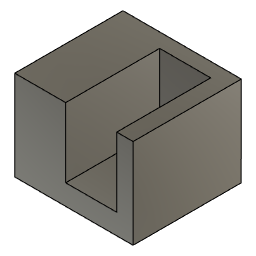
MotorHolder (Autodesk Fusion 360 design; units mm, degrees)
Autodesk Fusion 360 part; units mm, degrees
sketch "Sketch1" plane through (0, 0, 0) normal (0, 0, 1) x (1, 0, 0)
  line L0 (0, 0) -> (17, 0)
  line L1 (17, 0) -> (17, 23)
  line L2 (17, 23) -> (0, 23)
  line L3 (0, 23) -> (0, 0)
  dimension "d1" = 17
  dimension "d2" = 23
  constraint horizontal L0
  constraint vertical L1
  constraint horizontal L2
  constraint vertical L3
  constraint coincident L0.start L3.end
  measures "d1" distance of L0.start L0.end
  measures "d2" distance of L0.start L2.end
extrude "Extrude1" add sketch "Sketch1" along normal blind 3.5 makes body 1
sketch "Sketch2" plane through (0, 0, 3.5) normal (0, 0, 1) x (-1, 0, 0)
  line L0 (0, -23) -> (0, 0)
  line L1 (0, 0) -> (-17, 0)
  line L2 (-17, 0) -> (-17, -23)
  line L3 (-17, -23) -> (0, -23)
  line L4 (0, -25) -> (-17, -25)
  line L5 (-17, -25) -> (-17, -28.5)
  line L6 (-17, -28.5) -> (0, -28.5)
  line L7 (0, -28.5) -> (0, -25)
  dimension "d5" = 3.5
  constraint horizontal L4
  constraint vertical L5
  constraint horizontal L6
  constraint vertical L7
  measures "d5" distance of L4.start L6.end
extrude "Extrude2" add sketch "Sketch2" along normal blind 19 separate body contours L4 L5 L6 L7 makes body 2
copy_body "CopyPasteBodies1" bodies 1 makes body 3
move_body "Move1" bodies 3 to x (1, 0, 0) y (0, 1, 0) z (0, 0, 1) at (0, 0, 16)
move_body "Move2" bodies 2 to x (1, 0, 0) y (0, 1, 0) z (0, 0, 1) at (0, -2, -3.5)
move_body "Move3" bodies 3 to x (1, 0, 0) y (0, 1, 0) z (0, 0, 1) at (0, 0, -0.5)
sketch "Sketch3" plane through (0, 0, 0) normal (0, 1, 0) x (1, 0, 0)
sketch "Sketch4" plane through (0, 0, 0) normal (1, 0, 0) x (0, 1, 0)
  line L0 (26.467, 0.0177) -> (0, 0.0177)
  line L1 (0, 0.0177) -> (0, 19)
  line L2 (0, 19) -> (26.467, 19)
  line L3 (26.467, 19) -> (26.467, 0.0177)
  constraint horizontal L0
  constraint vertical L1
  constraint horizontal L2
  constraint vertical L3
move_body "Move4" bodies 3 2 1 to x (1, 0, 0) y (0, 1, 0) z (0, 0, 1) at (10, 0, 0)
extrude "Extrude3" add sketch "Sketch4" along normal blind 5 separate body makes body 4
move_body "Move5" bodies 4 to x (1, 0, 0) y (0, 1, 0) z (0, 0, 1) at (27, 0, 0)
combine "Combine1" operation add target body 2 tool bodies 3
combine "Combine2" operation add target body 2 tool bodies 1
combine "Combine3" operation add target body 4 tool bodies 2
move_body "Move6" bodies 4 to x (-1, 0, 0) y (0, 1, 0) z (0, 0, -1) at (56.1982, 0, 38)
move_body "Move7" bodies 4 to x (1, 0, 0) y (0, 1, 0) z (0, 0, 1) at (-19, 0, -19)
extrude "Extrude4" cut 1 faces at (21.5315, 15.3333, 3.5) along direction (0, 0, -1) blind 0.5 on bodies 4 bodies 4
extrude "Extrude5" cut 1 faces at (21.5315, 15.3333, 15.5) along direction (0, 0, 1) blind 0.5 on bodies 4 bodies 4
extrude "Extrude6" add 1 faces at (6.8648, 16.489, 18.9823) along direction (0, 0, 1) blind 10 on bodies 4 bodies 4
extrude "Extrude7" add 1 faces at (21.5315, 16.5, 19) along direction (0, 0, 1) blind 9.982 on bodies 4 bodies 4
move_body "Move8" bodies 4 to x (0, 0, 1) y (0, 1, 0) z (-1, 0, 0) at (43.779, 0, -1.7066)
move_body "Move9" bodies 4 to x (1, 0, 0) y (0, 1, 0) z (0, 0, 1) at (-14.25, 0, -3.5)
extrude "Extrude8" cut 1 faces at (13.529, 15.3333, 16.3249) along direction (-1, 0, 0) blind 0.5 on bodies 4 bodies 4
extrude "Extrude9" add 1 faces at (26.529, 15.3333, 16.3249) along direction (-1, 0, 0) blind 1 on bodies 4 bodies 4
